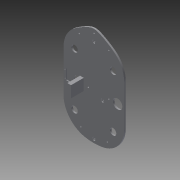
# Autodesk Inventor part: body
Saved by Autodesk Inventor 2014 (Build 180170000, 170)
## iProperties
Created: 2015-05-23
Part Number: body
Material: 一般
Document SubType Name: Modeling
Designer: Hideyuki Takei
Density: 1 g/cm^3
Appearance: 既定
d0: 115.000 mm
d1: 130.000 mm
d2: 65.000 mm
d3: 57.500 mm
d4: 3.000 mm
d5: 0.00 deg
d6: 12.200 mm
d7: 12.200 mm
d8: 12.200 mm
d9: 12.200 mm
d10: 21.000 mm
d11: 21.000 mm
d12: 15.000 mm
d13: 15.000 mm
d14: 15.000 mm
d15: 15.000 mm
d16: 21.000 mm
d17: 21.000 mm
d31: 3.000 mm
d32: 0.00 deg
d35: 0.000 mm
d36: 30.000 mm
d37: 17.000 mm
d38: 3.000 mm
d39: 0.00 deg
d40: 19.600 mm
d41: 15.700 mm
d42: 9.800 mm
d43: 7.000 mm
d44: 1.500 mm
d45: 0.00 deg
d46: 5.000 mm
d47: 1.000 mm
d48: 24.900 mm
d49: 24.900 mm
d50: 7.200 mm
d51: 7.200 mm
d53: 0.00 deg
d54: 2.100 mm
d55: 2.100 mm
d56: 3.600 mm
d57: 3.600 mm
d58: 2.000 mm
d59: 0.00 deg
d60: 19.600 mm
d61: 9.800 mm
d62: 2.000 mm
d63: 8.900 mm
d70: 5.050 mm
d71: 5.050 mm
d72: 5.050 mm
d73: 5.050 mm
d74: 22.200 mm
d75: 0.00 deg
d76: 10.100 mm
d77: 10.100 mm
d78: 22.200 mm
d79: 0.00 deg
d88: 1.000 mm
d89: 1.000 mm
d90: 7.050 mm
d91: 7.050 mm
d92: 2.000 mm
d93: 0.00 deg
d94: 30.000 mm
d95: 15.000 mm
d96: 15.000 mm
d97: 15.000 mm
d98: 15.000 mm
d99: 57.500 mm
d100: 3.000 mm
d101: 0.00 deg
d102: 0.000 mm
d103: 50.000 mm
d104: 11.000 mm
d105: 11.000 mm
d106: 25.000 mm
d107: 25.000 mm
d108: 33.000 mm
d109: 33.000 mm
d110: 38.000 mm
d111: 10.000 mm
d112: 10.000 mm
d113: 30.000 mm
d114: 30.000 mm
d115: 45.000 mm
d116: 45.000 mm
d117: 57.500 mm
d118: 3.000 mm
d119: 0.00 deg
d120: 50.000 mm
d123: 18.000 mm
d124: 0.000 mm
d125: 45.000 mm
d126: 3.000 mm
d127: 0.00 deg
d130: 5.000 mm
d131: 0.000 mm
d132: 8.660 mm
d133: 9.600 mm
d134: 0.00 deg
d135: 5.000 mm
d136: 0.000 mm
d137: 8.660 mm
d146: 0.000 mm
d147: 0.000 mm
d148: 27.273 mm
d149: 47.727 mm
d151: 5.000 mm
d152: 0.000 mm
d153: 0.000 mm
d154: 27.273 mm
d155: 27.273 mm
d156: 47.727 mm
d157: 5.000 mm
d158: 3.200 mm
d159: 79.800 mm
d160: 79.800 mm
d161: 3.200 mm
d162: 10.000 mm
d163: 0.00 deg
d164: 16.000 mm
d165: 9.000 mm
d166: 3.200 mm
d167: 5.600 mm
d169: 5.600 mm
d171: 5.600 mm
d173: 2.000 mm
d174: 0.00 deg
Author: Hideyuki Takei
Autodesk Inventor part; units mm, degrees
ref_plane "YZ Plane" through (0, 0, 0) normal (1, 0, 0) x (0, 1, 0)
ref_plane "XZ Plane" through (0, 0, 0) normal (0, 1, 0) x (-1, 0, 0)
ref_plane "XY Plane" through (0, 0, 0) normal (0, 0, 1) x (1, 0, 0)
sketch "スケッチ1" plane through (0, 0, 0) normal (0, 1, 0) x (-1, 0, 0)
  line L0 (-57.5, 65) -> (57.5, 65)
  line L1 (57.5, 65) -> (57.5, -65)
  line L2 (57.5, -65) -> (-57.5, -65)
  line L3 (-57.5, -65) -> (-57.5, 65)
  point P0 (0, 0)
  dimension "d0" = 115
  dimension "d1" = 130
  dimension "d2" = 65
  dimension "d3" = 57.5
  constraints: 8 end point, 2 parallel, 1 horizontal, 1 perpendicular
  measures "d0" distance of L0.start L0.end
  measures "d1" distance of L2.end L0.start
  measures "d2" distance from line of L0 point (0, 0)
  measures "d3" distance from line of point (0, 0) L3
extrude "押し出し1" add sketch "スケッチ1" along normal blind 3
sketch "スケッチ2" plane through (0, 3, 0) normal (0, 1, 0) x (1, 0, 0)
  line L0 (-57.5, -65) -> (57.5, -65) projected
  line L1 (57.5, -65) -> (57.5, 65) projected
  line L2 (57.5, 65) -> (-57.5, 65) projected
  line L3 (-57.5, 65) -> (-57.5, -65) projected
  circle A0 centre (-36.5, -50) radius 6.1
  circle A1 centre (36.5, -50) radius 6.1
  circle A2 centre (36.5, 50) radius 6.1
  circle A3 centre (-36.5, 50) radius 6.1
  dimension "d6" = 12.2
  dimension "d7" = 12.2
  dimension "d8" = 12.2
  dimension "d9" = 12.2
  dimension "d10" = 21
  dimension "d11" = 21
  dimension "d12" = 15
  dimension "d13" = 15
  dimension "d14" = 15
  dimension "d15" = 15
  dimension "d16" = 21
  dimension "d17" = 21
  constraints: 4 centre point
  measures "d6" diameter of A3
  measures "d7" diameter of A2
  measures "d8" diameter of A1
  measures "d9" diameter of A0
  measures "d10" distance from line of A0.centre L3
  measures "d11" distance from line of L1 A1.centre
  measures "d12" distance from line of L0 A0.centre
  measures "d13" distance from line of L0 A1.centre
  measures "d14" distance from line of L2 A2.centre
  measures "d15" distance from line of L2 A3.centre
  measures "d16" distance from line of L3 A3.centre
  measures "d17" distance from line of L1 A2.centre
extrude "押し出し4" cut sketch "スケッチ2" against normal blind 3 contours A0 | A1 | A2 | A3
sketch "スケッチ4" plane through (0, 0, 0) normal (0, 1, 0) x (-1, 0, 0)
  circle A0 centre (30, 0) radius 8.5
  point P0 (0, 0)
  dimension "d35" = 0
  dimension "d36" = 30
  dimension "d37" = 17
  constraints: 1 centre point
  measures "d35" vertical distance of A0.centre point (0, 0)
  measures "d36" distance of point (0, 0) A0.centre
  measures "d37" diameter of A0
extrude "押し出し5" cut sketch "スケッチ4" along normal blind 3
sketch "スケッチ7" plane through (0, 0, 0) normal (0, 1, 0) x (-1, 0, 0)
  line L0 (52.7, 9.8) -> (37, 9.8)
  line L1 (37, 9.8) -> (37, -9.8)
  line L2 (37, -9.8) -> (52.7, -9.8)
  line L3 (52.7, -9.8) -> (52.7, 9.8)
  circle A0 centre (30, 0) radius 8.5 projected
  point P0 (0, 0)
  dimension "d40" = 19.6
  dimension "d41" = 15.7
  dimension "d42" = 9.8
  dimension "d43" = 7
  constraints: 8 end point, 2 parallel, 1 horizontal, 1 perpendicular
  measures "d40" distance of L2.end L0.start
  measures "d41" distance of L0.start L0.end
  measures "d42" distance from line of point (0, 0) L0
  measures "d43" distance from line of A0.centre L1
extrude "押し出し6" cut sketch "スケッチ7" along normal blind 1.5 contours L3 L2 L1 A0 L0 | A0 L1 picked at (37.274, 1.1089)
fillet "フィレット1" radius 5 2 edges at (-37, 0.75, -9.8) (-37, 0.75, 9.8)
fillet "フィレット1" radius 1 2 edges at (-52.7, 0.75, -9.8) (-52.7, 0.75, 9.8)
sketch "スケッチ8" plane through (0, 0, 0) normal (0, 1, 0) x (-1, 0, 0)
  arc A0 (37, 4.8218) -> (37, -4.8218) centre (30, 0) ccw projected
  arc A1 (52.7, 8.8) -> (51.7, 9.8) centre (51.7, 8.8) ccw projected
  line L0 (52.7, -8.8) -> (52.7, 8.8) projected
  arc A2 (51.7, -9.8) -> (52.7, -8.8) centre (51.7, -8.8) ccw projected
  line L1 (42, -9.8) -> (51.7, -9.8) projected
  arc A3 (37, -4.8218) -> (42, -9.8) centre (42, -4.8) ccw projected
  arc A4 (37, -4.8218) -> (37, 4.8218) centre (30, 0) ccw projected
  arc A5 (42, 9.8) -> (37, 4.8218) centre (42, 4.8) ccw projected
  line L2 (51.7, 9.8) -> (42, 9.8) projected
  circle A6 centre (54.9, 7.2) radius 1.05
  circle A7 centre (54.9, -7.2) radius 1.05
  point P0 (0, 0)
  dimension "d48" = 24.9
  dimension "d49" = 24.9
  dimension "d50" = 7.2
  dimension "d51" = 7.2
  dimension "d54" = 2.1
  dimension "d55" = 2.1
  constraints: 2 centre point
  measures "d48" horizontal distance of A6.centre A0.centre
  measures "d49" horizontal distance of A0.centre A7.centre
  measures "d50" vertical distance of A6.centre A0.centre
  measures "d51" vertical distance of A7.centre A0.centre
  measures "d54" diameter of A6
  measures "d55" diameter of A7
extrude "押し出し7" cut sketch "スケッチ8" along normal up to next contours A6 | A7
sketch "スケッチ9" plane through (0, 3, 0) normal (0, 1, 0) x (1, 0, 0)
  circle A0 centre (-54.9, -7.2) radius 1.05 projected
  circle A1 centre (-54.9, 7.2) radius 1.05 projected
  circle A2 centre (-54.9, 7.2) radius 1.8
  circle A3 centre (-54.9, -7.2) radius 1.8
  point P0 (0, 0)
  dimension "d56" = 3.6
  dimension "d57" = 3.6
  constraints: 2 centre point, 2 coincident
  measures "d56" diameter of A2
  measures "d57" diameter of A3
extrude "押し出し8" cut sketch "スケッチ9" against normal blind 2
sketch "スケッチ10" plane through (0, 0, 0) normal (0, 1, 0) x (-1, 0, 0)
  line L0 (21.1, 9.8) -> (19.1, 9.8)
  line L1 (19.1, 9.8) -> (19.1, -9.8)
  line L2 (19.1, -9.8) -> (21.1, -9.8)
  line L3 (21.1, -9.8) -> (21.1, 9.8)
  arc A0 (37, 4.8218) -> (37, -4.8218) centre (30, 0) ccw projected
  arc A1 (42, 9.8) -> (37, 4.8218) centre (42, 4.8) ccw projected
  arc A2 (52.7, 8.8) -> (51.7, 9.8) centre (51.7, 8.8) ccw projected
  line L4 (52.7, -8.8) -> (52.7, 8.8) projected
  arc A3 (51.7, -9.8) -> (52.7, -8.8) centre (51.7, -8.8) ccw projected
  line L5 (42, -9.8) -> (51.7, -9.8) projected
  arc A4 (37, -4.8218) -> (42, -9.8) centre (42, -4.8) ccw projected
  arc A5 (37, -4.8218) -> (37, 4.8218) centre (30, 0) ccw projected
  arc A6 (42, 9.8) -> (37, 4.8218) centre (42, 4.8) ccw projected
  line L6 (51.7, 9.8) -> (42, 9.8) projected
  line L7 (21.1, 9.8) -> (26.15, 9.8)
  line L8 (26.15, 9.8) -> (26.15, 4.75)
  line L9 (26.15, 4.75) -> (21.1, 4.75)
  line L10 (21.1, 4.75) -> (21.1, 9.8)
  line L11 (21.1, -9.8) -> (26.15, -9.8)
  line L12 (26.15, -9.8) -> (26.15, -4.75)
  line L13 (26.15, -4.75) -> (21.1, -4.75)
  line L14 (21.1, -4.75) -> (21.1, -9.8)
  line L15 (26.15, 9.8) -> (19.1, 9.8)
  line L16 (19.1, 9.8) -> (19.1, 10.8)
  line L17 (19.1, 10.8) -> (26.15, 10.8)
  line L18 (26.15, 10.8) -> (26.15, 9.8)
  line L19 (26.15, -9.8) -> (19.1, -9.8)
  line L20 (19.1, -9.8) -> (19.1, -10.8)
  line L21 (19.1, -10.8) -> (26.15, -10.8)
  line L22 (26.15, -10.8) -> (26.15, -9.8)
  point P0 (0, 0)
  dimension "d94" = 30
  dimension "d60" = 19.6
  dimension "d61" = 9.8
  dimension "d62" = 2
  dimension "d63" = 8.9
  dimension "d70" = 5.05
  dimension "d71" = 5.05
  dimension "d72" = 5.05
  dimension "d73" = 5.05
  dimension "d88" = 1
  dimension "d89" = 1
  dimension "d90" = 7.05
  dimension "d91" = 7.05
  constraints: 40 end point, 10 parallel, 5 horizontal, 5 perpendicular
  measures "d60" distance of L0.end L1.end
  measures "d61" distance from line of point (0, 0) L0
  measures "d62" distance of L0.start L0.end
  measures "d63" distance from line of L3 A0.centre
  measures "d70" distance of L7.end L8.end
  measures "d71" distance of L8.end L9.end
  measures "d72" distance of L11.end L12.end
  measures "d73" distance of L12.end L13.end
  measures "d88" distance of L19.end L20.end
  measures "d89" distance of L15.end L16.end
  measures "d90" distance of L16.end L17.end
  measures "d91" distance of L20.end L21.end
extrude "押し出し9" add sketch "スケッチ10" against normal blind 22.2 contours L3 L2 L1 L0 | L7 L8 A0 L9 L3 | L0 L16 L17 L18 L7 | L2 L11 L22 L21 L20 | L13 A0 L12 L11 L3 | A0 L8 L9 | L13 L12 A0
sketch "スケッチ11" plane through (0, 0, 0) normal (0, 1, 0) x (-1, 0, 0)
  arc A0 (37, 4.8218) -> (37, -4.8218) centre (30, 0) ccw projected
  arc A1 (52.7, 8.8) -> (51.7, 9.8) centre (51.7, 8.8) ccw projected
  line L0 (52.7, -8.8) -> (52.7, 8.8) projected
  arc A2 (51.7, -9.8) -> (52.7, -8.8) centre (51.7, -8.8) ccw projected
  line L1 (42, -9.8) -> (51.7, -9.8) projected
  arc A3 (37, -4.8218) -> (42, -9.8) centre (42, -4.8) ccw projected
  arc A4 (37, -4.8218) -> (37, 4.8218) centre (30, 0) ccw projected
  arc A5 (42, 9.8) -> (37, 4.8218) centre (42, 4.8) ccw projected
  line L2 (51.7, 9.8) -> (42, 9.8) projected
  line L3 (19.1, -10.8) -> (19.1, 10.8) projected
  line L4 (26.15, 10.8) -> (26.15, 4.75) projected
  line L5 (26.15, 4.75) -> (21.1, 4.75) projected
  line L6 (21.1, 4.75) -> (21.1, -4.75) projected
  line L7 (21.1, -4.75) -> (26.15, -4.75) projected
  line L8 (26.15, -4.75) -> (26.15, -10.8) projected
  circle A6 centre (26.15, 4.75) radius 5.05
  circle A7 centre (26.15, -4.75) radius 5.05
  line L9 (19.1, 10.8) -> (26.15, 10.8) projected
  line L10 (26.15, -10.8) -> (19.1, -10.8) projected
  point P0 (0, 0)
  dimension "d76" = 10.1
  dimension "d77" = 10.1
  constraints: 2 centre point, 2 coincident
  measures "d76" diameter of A6
  measures "d77" diameter of A7
extrude "押し出し10" cut sketch "スケッチ11" against normal blind 22.2 contours A6 A7 A0 L5 L4 | A0 L4 A6 | L4 L5 A0 | A0 L5 A6 L4 | A7 L8 A0 | A0 L8 L7 A7 A6 | A0 A6 L5 | A6 A7 | L8 A7 L7 A0 | A0 L7 L8 | A7 A0 L7
sketch "スケッチ14" plane through (0, -22.2, 0) normal (0, -1, 0) x (1, 0, 0)
  line L0 (-19.1, 10.8) -> (-26.15, 10.8)
  line L1 (-26.15, 10.8) -> (-26.15, -10.8)
  line L2 (-26.15, -10.8) -> (-19.1, -10.8)
  line L3 (-19.1, -10.8) -> (-19.1, 10.8)
  point P0 (0, 0)
  constraints: 8 end point, 2 parallel, 1 horizontal, 1 perpendicular
extrude "押し出し13" add sketch "スケッチ14" along normal blind 2
sketch "スケッチ15" plane through (0, 0, 0) normal (0, 1, 0) x (-1, 0, 0)
  line L0 (26.15, 9.8) -> (26.15, 10.8) projected
  line L1 (26.15, 10.8) -> (19.1, 10.8) projected
  line L2 (19.1, 10.8) -> (19.1, -10.8) projected
  line L3 (19.1, -10.8) -> (26.15, -10.8) projected
  line L4 (26.15, -10.8) -> (26.15, -9.8) projected
  arc A0 (21.1, -4.75) -> (26.15, -9.8) centre (26.15, -4.75) ccw projected
  line L5 (21.1, -4.75) -> (21.1, 4.75) projected
  arc A1 (26.15, 9.8) -> (21.1, 4.75) centre (26.15, 4.75) ccw projected
  circle A2 centre (-36.5, -50) radius 6.1 projected
  circle A3 centre (36.5, 50) radius 6.1 projected
  circle A4 centre (-36.5, 50) radius 6.1 projected
  circle A5 centre (36.5, -50) radius 6.1 projected
  line L6 (-57.5, 65) -> (57.5, 65) projected
  line L7 (57.5, 65) -> (57.5, -65) projected
  line L8 (57.5, -65) -> (-57.5, -65) projected
  line L9 (-57.5, -65) -> (-57.5, 65) projected
  circle A6 centre (54.9, -7.2) radius 1.05 projected
  circle A7 centre (54.9, 7.2) radius 1.05 projected
  arc A8 (37, 4.8218) -> (37, -4.8218) centre (30, 0) ccw projected
  arc A9 (37, -4.8218) -> (42, -9.8) centre (42, -4.8) ccw projected
  line L10 (42, -9.8) -> (51.7, -9.8) projected
  arc A10 (51.7, -9.8) -> (52.7, -8.8) centre (51.7, -8.8) ccw projected
  line L11 (52.7, -8.8) -> (52.7, 8.8) projected
  arc A11 (52.7, 8.8) -> (51.7, 9.8) centre (51.7, 8.8) ccw projected
  line L12 (51.7, 9.8) -> (42, 9.8) projected
  arc A12 (42, 9.8) -> (37, 4.8218) centre (42, 4.8) ccw projected
  line L13 (57.5, -65) -> (57.5, -65) construction
  line L14 (57.5, -65) -> (42.5, -80) construction
  line L15 (42.5, -80) -> (0, -95) construction
  line L16 (0, -95) -> (-42.5, -80) construction
  line L17 (-42.5, -80) -> (-57.5, -65) construction
  line L18 (-57.5, -65) -> (-57.5, -65) construction
  spline S0 degree 4 poles (57.5, -65) (57.485, -65.015) (42.5, -80) (0, -95) (-42.5, -80) (-57.485, -65.015) (-57.5, -65) knots 1 1 1 1 1 2 3 4 4 4 4 4
  line L19 (57.5, -65) -> (-57.5, -65)
  point P0 (0, 0)
  dimension "d94" = 30
  dimension "d95" = 15
  dimension "d96" = 15
  dimension "d97" = 15
  dimension "d98" = 15
  dimension "d99" = 57.5
  dimension "d102" = 0
  constraints: 2 coincident, 2 collinear, 2 end point, 2 point on line, 3 other
  measures "d94" distance from line of L8 L15.end
  measures "d95" distance from line of L8 L16.end
  measures "d96" distance from line of L8 L14.end
  measures "d97" horizontal distance of L18.end L16.end
  measures "d98" horizontal distance of L13.start L14.end
  measures "d99" horizontal distance of L13.start L15.end
  measures "d102" distance between parallel lines of L19 L8
extrude "押し出し14" add sketch "スケッチ15" along normal blind 3 contours L8 S0
fillet "フィレット2" radius 50 2 edges at (-57.5, 1.5, -65) (57.5, 1.5, -65)
sketch "スケッチ16" plane through (0, 0, 0) normal (0, 1, 0) x (-1, 0, 0)
  line L0 (26.15, 9.8) -> (26.15, 10.8) projected
  line L1 (26.15, 10.8) -> (19.1, 10.8) projected
  line L2 (19.1, 10.8) -> (19.1, -10.8) projected
  line L3 (19.1, -10.8) -> (26.15, -10.8) projected
  line L4 (26.15, -10.8) -> (26.15, -9.8) projected
  arc A0 (21.1, -4.75) -> (26.15, -9.8) centre (26.15, -4.75) ccw projected
  line L5 (21.1, -4.75) -> (21.1, 4.75) projected
  arc A1 (26.15, 9.8) -> (21.1, 4.75) centre (26.15, 4.75) ccw projected
  circle A2 centre (-36.5, -50) radius 6.1 projected
  circle A3 centre (36.5, 50) radius 6.1 projected
  circle A4 centre (-36.5, 50) radius 6.1 projected
  circle A5 centre (36.5, -50) radius 6.1 projected
  line L6 (-57.5, -36.0771) -> (-57.5, 65) projected
  line L7 (-57.5, 65) -> (57.5, 65) projected
  line L8 (57.5, 65) -> (57.5, -36.0771) projected
  circle A6 centre (54.9, -7.2) radius 1.05 projected
  circle A7 centre (54.9, 7.2) radius 1.05 projected
  arc A8 (37, 4.8218) -> (37, -4.8218) centre (30, 0) ccw projected
  arc A9 (37, -4.8218) -> (42, -9.8) centre (42, -4.8) ccw projected
  line L9 (42, -9.8) -> (51.7, -9.8) projected
  arc A10 (51.7, -9.8) -> (52.7, -8.8) centre (51.7, -8.8) ccw projected
  line L10 (52.7, -8.8) -> (52.7, 8.8) projected
  arc A11 (52.7, 8.8) -> (51.7, 9.8) centre (51.7, 8.8) ccw projected
  line L11 (51.7, 9.8) -> (42, 9.8) projected
  arc A12 (42, 9.8) -> (37, 4.8218) centre (42, 4.8) ccw projected
  line L12 (57.5, 65) -> (47.5, 76) construction
  line L13 (47.5, 76) -> (27.5, 90) construction
  line L14 (27.5, 90) -> (12.5, 98) construction
  line L15 (12.5, 98) -> (0, 103) construction
  line L16 (0, 103) -> (-12.5, 98) construction
  line L17 (-12.5, 98) -> (-27.5, 90) construction
  line L18 (-27.5, 90) -> (-47.5, 76) construction
  line L19 (-47.5, 76) -> (-57.5, 65) construction
  spline S0 degree 4 poles (57.5, 65) (47.5, 76) (27.5, 90) (12.5, 98) (0, 103) (-12.5, 98) (-27.5, 90) (-47.5, 76) (-57.5, 65) knots 0 0 0 0 0 1 2 3 4 5 5 5 5 5
  line L20 (57.5, 65) -> (-57.5, 65)
  point P0 (0, 0)
  dimension "d104" = 11
  dimension "d105" = 11
  dimension "d106" = 25
  dimension "d107" = 25
  dimension "d108" = 33
  dimension "d109" = 33
  dimension "d110" = 38
  dimension "d111" = 10
  dimension "d112" = 10
  dimension "d113" = 30
  dimension "d114" = 30
  dimension "d115" = 45
  dimension "d116" = 45
  dimension "d117" = 57.5
  constraints: 2 end point, 1 horizontal alignment, 1 parallel, 5 other
  measures "d104" distance from line of L7 L12.end
  measures "d105" distance from line of L7 L18.end
  measures "d106" distance from line of L7 L17.end
  measures "d107" distance from line of L7 L13.end
  measures "d108" distance from line of L7 L14.end
  measures "d109" distance from line of L7 L16.end
  measures "d110" distance from line of L7 L15.end
  measures "d111" distance from line of L8 L12.end
  measures "d112" distance from line of L6 L18.end
  measures "d113" distance from line of L17.end L6
  measures "d114" distance from line of L8 L13.end
  measures "d115" distance from line of L14.end L8
  measures "d116" distance from line of L6 L16.end
  measures "d117" distance from line of L8 L15.end
extrude "押し出し15" add sketch "スケッチ16" along normal blind 3 contours S0 L7
fillet "フィレット3" radius 50 2 edges at (-57.5, 1.5, 65) (57.5, 1.5, 65)
sketch "スケッチ17" plane through (0, 0, 0) normal (0, 1, 0) x (-1, 0, 0)
  line L0 (57.5, 42.5858) -> (57.5, -36.0771) projected
  line L1 (-57.5, -36.0771) -> (-57.5, 42.5858) projected
  line L2 (26.15, 9.8) -> (26.15, 10.8) projected
  line L3 (26.15, 10.8) -> (19.1, 10.8) projected
  line L4 (19.1, 10.8) -> (19.1, -10.8) projected
  line L5 (19.1, -10.8) -> (26.15, -10.8) projected
  line L6 (26.15, -10.8) -> (26.15, -9.8) projected
  arc A0 (21.1, -4.75) -> (26.15, -9.8) centre (26.15, -4.75) ccw projected
  line L7 (21.1, -4.75) -> (21.1, 4.75) projected
  arc A1 (26.15, 9.8) -> (21.1, 4.75) centre (26.15, 4.75) ccw projected
  circle A2 centre (-36.5, -50) radius 6.1 projected
  circle A3 centre (36.5, 50) radius 6.1 projected
  circle A4 centre (-36.5, 50) radius 6.1 projected
  circle A5 centre (36.5, -50) radius 6.1 projected
  circle A6 centre (54.9, -7.2) radius 1.05 projected
  circle A7 centre (54.9, 7.2) radius 1.05 projected
  arc A8 (37, 4.8218) -> (37, -4.8218) centre (30, 0) ccw projected
  arc A9 (37, -4.8218) -> (42, -9.8) centre (42, -4.8) ccw projected
  line L8 (42, -9.8) -> (51.7, -9.8) projected
  arc A10 (51.7, -9.8) -> (52.7, -8.8) centre (51.7, -8.8) ccw projected
  line L9 (52.7, -8.8) -> (52.7, 8.8) projected
  arc A11 (52.7, 8.8) -> (51.7, 9.8) centre (51.7, 8.8) ccw projected
  line L10 (51.7, 9.8) -> (42, 9.8) projected
  arc A12 (42, 9.8) -> (37, 4.8218) centre (42, 4.8) ccw projected
  circle A13 centre (-45, 0) radius 9
  point P0 (0, 0)
  dimension "d123" = 18
  dimension "d124" = 0
  dimension "d125" = 45
  constraints: 2 horizontal alignment, 1 centre point, 4 other
  measures "d123" diameter of A13
  measures "d124" vertical distance of point (0, 0) A13.centre
  measures "d125" distance of point (0, 0) A13.centre
extrude "押し出し16" cut sketch "スケッチ17" along normal blind 3 contours A13
sketch "スケッチ19" plane through (0, 0, 0) normal (0, 1, 0) x (-1, 0, 0)
  circle A0 centre (-45, 0) radius 9 projected
  line L0 (57.5, 42.5858) -> (57.5, -36.0771) projected
  line L1 (-57.5, -36.0771) -> (-57.5, 42.5858) projected
  line L2 (26.15, 9.8) -> (26.15, 10.8) projected
  line L3 (26.15, 10.8) -> (19.1, 10.8) projected
  line L4 (19.1, 10.8) -> (19.1, -10.8) projected
  line L5 (19.1, -10.8) -> (26.15, -10.8) projected
  line L6 (26.15, -10.8) -> (26.15, -9.8) projected
  arc A1 (21.1, -4.75) -> (26.15, -9.8) centre (26.15, -4.75) ccw projected
  line L7 (21.1, -4.75) -> (21.1, 4.75) projected
  arc A2 (26.15, 9.8) -> (21.1, 4.75) centre (26.15, 4.75) ccw projected
  circle A3 centre (-36.5, -50) radius 6.1 projected
  circle A4 centre (36.5, 50) radius 6.1 projected
  circle A5 centre (-36.5, 50) radius 6.1 projected
  circle A6 centre (36.5, -50) radius 6.1 projected
  circle A7 centre (54.9, -7.2) radius 1.05 projected
  circle A8 centre (54.9, 7.2) radius 1.05 projected
  arc A9 (37, 4.8218) -> (37, -4.8218) centre (30, 0) ccw projected
  arc A10 (37, -4.8218) -> (42, -9.8) centre (42, -4.8) ccw projected
  line L8 (42, -9.8) -> (51.7, -9.8) projected
  arc A11 (51.7, -9.8) -> (52.7, -8.8) centre (51.7, -8.8) ccw projected
  line L9 (52.7, -8.8) -> (52.7, 8.8) projected
  arc A12 (52.7, 8.8) -> (51.7, 9.8) centre (51.7, 8.8) ccw projected
  line L10 (51.7, 9.8) -> (42, 9.8) projected
  arc A13 (42, 9.8) -> (37, 4.8218) centre (42, 4.8) ccw projected
  circle A14 centre (0, 41.34) radius 2.5
  circle A15 centre (0, -41.34) radius 2.5
  circle A16 centre (30, 0) radius 13.6364
  circle A17 centre (3.0165, -3.9615) radius 13.6364
  circle A18 centre (0, -41.34) radius 23.8636
  circle A19 centre (3.0165, -3.9615) radius 2.5
  circle A20 centre (0, 41.34) radius 23.8636
  circle A21 centre (-20.4622, 9.9147) radius 13.6364
  circle A22 centre (-20.4622, 9.9147) radius 2.5
  point P0 (0, 0)
  point P1 (0.747, -2.0638)
  dimension "d130" = 5
  dimension "d131" = 0
  dimension "d132" = 8.66
  dimension "d135" = 5
  dimension "d136" = 0
  dimension "d137" = 8.66
  dimension "d146" = 0
  dimension "d147" = 0
  dimension "d148" = 27.2727
  dimension "d149" = 47.7273
  dimension "d151" = 5
  dimension "d152" = 0
  dimension "d153" = 0
  dimension "d154" = 27.2727
  dimension "d155" = 27.2727
  dimension "d156" = 47.7273
  dimension "d157" = 5
  constraints: 9 centre point, 5 coincident, 2 horizontal alignment, 4 other
  measures "d130" diameter of A14
  measures "d131" horizontal distance of point (0, 0) A14.centre
  measures "d132" vertical distance of A4.centre A14.centre
  measures "d135" diameter of A15
  measures "d136" horizontal distance of point (0, 0) A15.centre
  measures "d137" vertical distance of A6.centre A15.centre
  measures "d148" diameter of A16
  measures "d149" diameter of A18
  measures "d151" diameter of A19
  measures "d154" diameter of A17
  measures "d155" diameter of A21
  measures "d156" diameter of A20
  measures "d157" diameter of A22
extrude "押し出し17" add sketch "スケッチ19" along normal blind 9.6 contours A14 | A15 | A19 | A22
sketch "スケッチ20" plane through (0, 0, 0) normal (0, 1, 0) x (-1, 0, 0)
  circle A0 centre (0, 79.8) radius 1.6
  circle A1 centre (0, -79.8) radius 1.6
  circle A2 centre (-16, -9) radius 1.6
  point P0 (0, 0)
  dimension "d158" = 3.2
  dimension "d159" = 79.8
  dimension "d160" = 79.8
  dimension "d161" = 3.2
  dimension "d164" = 16
  dimension "d165" = 9
  dimension "d166" = 3.2
  constraints: 3 centre point
  measures "d158" diameter of A1
  measures "d159" distance of A1.centre point (0, 0)
  measures "d160" distance of A0.centre point (0, 0)
  measures "d161" diameter of A0
  measures "d164" horizontal distance of A2.centre point (0, 0)
  measures "d165" vertical distance of A2.centre point (0, 0)
  measures "d166" diameter of A2
extrude "押し出し18" cut sketch "スケッチ20" along normal blind 10
sketch "スケッチ21" plane through (0, 0, 0) normal (0, 1, 0) x (-1, 0, 0)
  circle A0 centre (0, 79.8) radius 1.6 projected
  circle A1 centre (-16, -9) radius 1.6 projected
  circle A2 centre (0, -79.8) radius 1.6 projected
  line L0 (-3.2331, 79.7892) -> (-1.6259, 82.5946)
  line L1 (-1.6259, 82.5946) -> (1.6072, 82.6054)
  line L2 (1.6072, 82.6054) -> (3.2331, 79.8108)
  line L3 (3.2331, 79.8108) -> (1.6259, 77.0054)
  line L4 (1.6259, 77.0054) -> (-1.6072, 76.9946)
  line L5 (-1.6072, 76.9946) -> (-3.2331, 79.7892)
  line L6 (-19.2332, -9) -> (-17.6166, -6.2)
  line L7 (-17.6166, -6.2) -> (-14.3834, -6.2)
  line L8 (-14.3834, -6.2) -> (-12.7668, -9)
  line L9 (-12.7668, -9) -> (-14.3834, -11.8)
  line L10 (-14.3834, -11.8) -> (-17.6166, -11.8)
  line L11 (-17.6166, -11.8) -> (-19.2332, -9)
  line L12 (-3.2332, -79.8) -> (-1.6166, -77)
  line L13 (-1.6166, -77) -> (1.6166, -77)
  line L14 (1.6166, -77) -> (3.2332, -79.8)
  line L15 (3.2332, -79.8) -> (1.6166, -82.6)
  line L16 (1.6166, -82.6) -> (-1.6166, -82.6)
  line L17 (-1.6166, -82.6) -> (-3.2332, -79.8)
  point P0 (0, 0)
  dimension "d167" = 5.6
  dimension "d169" = 5.6
  dimension "d171" = 5.6
  constraints: 36 end point, 6 coincident, 1 horizontal alignment, 39 other
  measures "d167" distance between parallel lines of L16 L13
  measures "d169" distance between parallel lines of L10 L7
  measures "d171" distance between parallel lines of L4 L1
extrude "押し出し19" cut sketch "スケッチ21" along normal blind 2
sketch "スケッチ22" plane through (0, 0, 0) normal (0, 1, 0) x (-1, 0, 0)
  circle A0 centre (0, 93.939) radius 1.6
  point P0 (0, 0)
  dimension "d177" = 3.2
  dimension "d178" = 93.939
  constraints: 1 centre point
  measures "d177" diameter of A0
  measures "d178" distance of A0.centre point (0, 0)
extrude "押し出し20" cut sketch "スケッチ22" along normal blind 10
sketch "スケッチ23" plane through (0, 0, 0) normal (0, 1, 0) x (-1, 0, 0)
  circle A0 centre (0, 79.8) radius 1.6 projected
  circle A1 centre (28, 79.8) radius 1.6
  circle A2 centre (-28, 79.8) radius 1.6
  circle A3 centre (25, -72) radius 1.6
  circle A4 centre (-25, -72) radius 1.6
  circle A5 centre (11, 0) radius 1.6
  circle A6 centre (-28, 0) radius 1.6
  point P0 (0, 0)
  dimension "d181" = 0
  dimension "d182" = 0
  dimension "d183" = 28
  dimension "d184" = 28
  dimension "d185" = 3.2
  dimension "d186" = 3.2
  dimension "d187" = 3.2
  dimension "d188" = 3.2
  dimension "d189" = 25
  dimension "d190" = 25
  dimension "d191" = 72
  dimension "d192" = 72
  dimension "d201" = 3.2
  dimension "d202" = 3.2
  dimension "d203" = 11
  dimension "d204" = 28
  constraints: 6 centre point
  measures "d181" vertical distance of A0.centre A1.centre
  measures "d182" vertical distance of A0.centre A2.centre
  measures "d183" distance of A0.centre A1.centre
  measures "d184" distance of A0.centre A2.centre
  measures "d185" diameter of A2
  measures "d186" diameter of A1
  measures "d187" diameter of A3
  measures "d188" diameter of A4
  measures "d189" horizontal distance of A3.centre point (0, 0)
  measures "d190" horizontal distance of point (0, 0) A4.centre
  measures "d191" vertical distance of A3.centre point (0, 0)
  measures "d192" vertical distance of point (0, 0) A4.centre
  measures "d201" diameter of A5
  measures "d202" diameter of A6
  measures "d203" distance of A5.centre point (0, 0)
  measures "d204" distance of point (0, 0) A6.centre
extrude "押し出し21" cut sketch "スケッチ23" along normal blind 10 contours A1 | A2 | A3 | A4 | A5 | A6
sketch "スケッチ24" plane through (0, 3, 0) normal (0, 1, 0) x (1, 0, 0)
  circle A0 centre (-25, 72) radius 1.6 projected
  circle A1 centre (-28, -79.8) radius 1.6 projected
  circle A2 centre (28, -79.8) radius 1.6 projected
  circle A3 centre (25, 72) radius 1.6 projected
  circle A4 centre (-25, 72) radius 3
  circle A5 centre (25, 72) radius 3
  circle A6 centre (-28, -79.8) radius 3
  circle A7 centre (28, -79.8) radius 3
  circle A8 centre (-11, 0) radius 1.6 projected
  circle A9 centre (28, 0) radius 1.6 projected
  circle A10 centre (-11, 0) radius 3
  circle A11 centre (28, 0) radius 3
  point P0 (0, 0)
  dimension "d195" = 6
  dimension "d196" = 6
  dimension "d197" = 6
  dimension "d198" = 6
  dimension "d205" = 6
  dimension "d206" = 6
  constraints: 6 centre point, 6 coincident
  measures "d195" diameter of A6
  measures "d196" diameter of A7
  measures "d197" diameter of A5
  measures "d198" diameter of A4
  measures "d205" diameter of A10
  measures "d206" diameter of A11
extrude "押し出し22" cut sketch "スケッチ24" against normal blind 1.5
equation "\"d2\" = 0.5 * d1"
equation "\"d3\" = 0.5 * d0"
equation "\"d6\" = d9"
equation "\"d7\" = d9"
equation "\"d8\" = d9"
equation "\"d42\" = 0.5 * d40"
equation "\"d49\" = d48"
equation "\"d51\" = d50"
equation "\"d55\" = d54"
equation "\"d61\" = 0.5 * d60"
equation "\"d72\" = d71"
equation "\"d73\" = d70"
equation "\"d137\" = d132"
equation "\"d160\" = d159"
equation "\"d161\" = d158"
equation "\"d166\" = d158"
equation "\"d184\" = d183"
equation "\"d190\" = d189"
equation "\"d192\" = d191"
